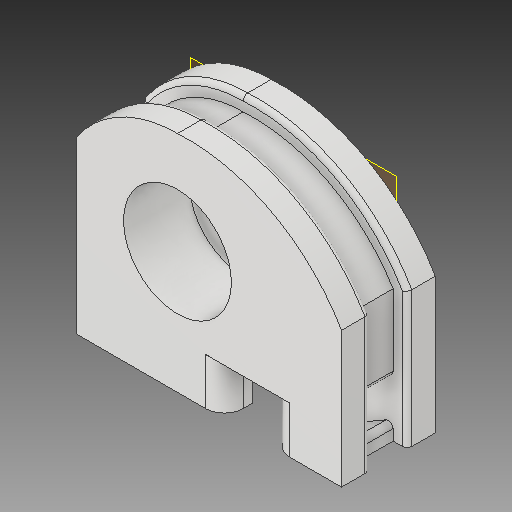
# Autodesk Inventor part: Gankenkunアンテナパーツ
Saved by Autodesk Inventor 2018 (Build 220112000, 112)
## iProperties
Category: コックピット
Created: 2018-04-09
Part Number: Gankenkunアンテナパーツ
Material: ABS プラスチック
Document SubType Name: Modeling
Designer: ito 017
Density: 1.06 g/cm^3
Appearance: 滑らか - 白
Author: ito 017
Autodesk Inventor part; units mm, degrees
ref_plane "YZ Plane" through (0, 0, 0) normal (1, 0, 0) x (0, 1, 0)
ref_plane "XZ Plane" through (0, 0, 0) normal (0, 1, 0) x (-1, 0, 0)
ref_plane "XY Plane" through (0, 0, 0) normal (0, 0, 1) x (1, 0, 0)
ref_plane "作業平面12" through (0, 0, 10) normal (0, 0, 1) x (1, 0, 0)
sketch "スケッチ48" plane through (0, 0, 10) normal (0, 0, 1) x (1, 0, 0)
  line L0 (-10.75, -3) -> (-10.75, 15.2244) projected
  line L1 (-10.75, -3) -> (17.5, -3)
  line L2 (17.5, -3) -> (17.5, 11.485)
  line L3 (-10.75, 11.485) -> (-10.75, -3)
  arc A0 (17.5, 11.485) -> (0, 20.9143) centre (1.069, 1.9444) ccw projected
  arc A1 (0, 20.9143) -> (-10.75, 15.2244) centre (0, 7.9143) ccw
  arc A2 (17.5, 11.485) -> (0, 20.9143) centre (1.069, 1.9444) ccw
  line L4 (-10.75, 15.2244) -> (-10.75, 11.485)
  circle A3 centre (0, 10) radius 3.5 projected
  circle A4 centre (0, 10) radius 3.5
  circle A5 centre (0, 10) radius 5.75
  point P0 (0, 0)
  constraints: 8 end point, 4 centre point, 4 point on circle, 2 coincident, 1 concentric, 1 horizontal, 1 parallel, 1 perpendicular, 1 vertical
extrude "押し出し40" add sketch "スケッチ48" along normal blind 10 contours L0 A1 A0 L2 L1 | A5
sketch "スケッチ50" plane through (0, 0, 20) normal (0, 0, 1) x (1, 0, 0)
  line L0 (-10.75, -3) -> (17.5, -3) projected
  line L1 (5, -3) -> (10, -3)
  line L2 (10, -3) -> (10, 2)
  line L3 (10, 2) -> (5, 2)
  line L4 (5, 2) -> (5, -3)
  line L5 (-10.75, 15.2244) -> (-10.75, -3) projected
  point P0 (0, 0)
  dimension "d179" = 15.75
  dimension "d180" = 5
  dimension "d181" = 5
  constraints: 8 end point, 2 parallel, 1 horizontal, 1 perpendicular, 1 point on line
  measures "d179" distance between parallel lines of L5 L4
  measures "d180" distance between parallel lines of L4 L2
  measures "d181" distance of L1.end L2.end
extrude "押し出し41" cut sketch "スケッチ50" against normal blind 10
sketch "スケッチ51" plane through (0, 0, 20) normal (0, 0, 1) x (1, 0, 0)
  circle A0 centre (0, 10) radius 5.75
  circle A1 centre (0, 10) radius 3.5 projected
  point P0 (0, 0)
  dimension "d184" = 11.5
  constraints: 1 centre point, 1 concentric
  measures "d184" diameter of A0
extrude "押し出し42" cut sketch "スケッチ51" against normal blind 7
sketch "スケッチ52" plane through (0, 0, 20) normal (0, 0, 1) x (1, 0, 0)
  line L0 (10, -3) -> (17.5, -3) projected
  line L1 (17.5, -3) -> (16, -3)
  line L2 (16, -3) -> (16, 11.0771)
  line L3 (16, 11.0771) -> (17.5, 11.0771)
  line L4 (17.5, 11.0771) -> (17.5, -3)
  line L5 (-10.75, -3) -> (5, -3) projected
  line L6 (-10.75, -3) -> (-9.25, -3)
  line L7 (-9.25, -3) -> (-9.25, 14.7471)
  line L8 (-9.25, 14.7471) -> (-10.75, 14.7471)
  line L9 (-10.75, 14.7471) -> (-10.75, -3)
  arc A0 (0, 20.9143) -> (-10.75, 15.2244) centre (0, 7.9143) ccw projected
  line L10 (0, 20.9143) -> (0, 19.4143)
  arc A1 (0, 19.4143) -> (-9.25, 14.7471) centre (0, 7.9143) ccw
  arc A2 (16, 11.0771) -> (0, 19.4143) centre (1.069, 1.9444) ccw
  arc A3 (17.5, 11.485) -> (0, 20.9143) centre (1.069, 1.9444) ccw projected
  line L11 (-10.75, 15.2244) -> (-10.75, 14.7471)
  line L12 (-10.75, 15.2244) -> (-10.75, -3) projected
  line L13 (17.5, -3) -> (17.5, 11.485) projected
  line L14 (17.5, 11.0771) -> (17.5, 11.485)
  point P0 (0, 0)
  dimension "d187" = 1.5
  dimension "d188" = 1.5
  dimension "d189" = 1.5
  constraints: 22 end point, 4 parallel, 4 point on circle, 2 centre point, 2 collinear, 2 concentric, 2 horizontal, 2 perpendicular, 1 vertical
  measures "d187" distance between parallel lines of L9 L7
  measures "d188" distance between parallel lines of L4 L2
  measures "d189" distance of L10.start L10.end
extrude "押し出し43" cut sketch "スケッチ52" against normal blind 7
sketch "スケッチ53" plane through (0, 0, 20) normal (0, 0, 1) x (1, 0, 0)
  line L0 (10, -3) -> (12.5, -3)
  line L1 (12.5, -3) -> (12.5, 0)
  line L2 (12.5, 0) -> (10, 0)
  line L3 (10, 0) -> (10, -3)
  line L4 (-10.75, -3) -> (5, -3) projected
  line L5 (5, -3) -> (0, -3)
  line L6 (0, -3) -> (0, -1)
  line L7 (0, -1) -> (5, -1)
  line L8 (5, -1) -> (5, -3)
  line L9 (12.5, -3) -> (16, -0.9793)
  line L10 (16, -3) -> (16, 11.0771) projected
  line L11 (10, 2) -> (10, -3) projected
  line L12 (10, -0.2865) -> (16, 3.1776)
  line L13 (10, -3) -> (16, -3) projected
  line L14 (0, -3) -> (-9.25, 2.382)
  line L15 (-9.25, 14.7471) -> (-9.25, -3) projected
  line L16 (5, -3) -> (5, 2) projected
  line L17 (5, -1.6285) -> (-9.25, 6.6628)
  point P0 (0, 0)
  dimension "d192" = 2.5
  dimension "d193" = 3
  dimension "d194" = 2
  dimension "d195" = 5
  dimension "d197" = 3.6
  dimension "d198" = 30
  dimension "d199" = 3.7
  constraints: 24 end point, 6 parallel, 6 point on line, 2 horizontal, 2 perpendicular
  measures "d192" distance of L0.start L0.end
  measures "d193" distance of L0.end L1.end
  measures "d194" distance of L5.end L6.end
  measures "d195" distance of L6.end L7.end
  measures "d197" distance between parallel lines of L9 L12
  measures "d198" angle of L13 L9
  measures "d199" distance between parallel lines of L17 L14
extrude "押し出し44" cut sketch "スケッチ53" against normal blind 7 contours L3 L12 L2 L1 L0 | L1 L2 L12 L10 L9 | L3 L2 L12 | L6 L7 L17 L8 L4 | L14 L15 L17 L7 L6 | L17 L7 L8
sketch "スケッチ54" plane through (0, 0, 20) normal (0, 0, 1) x (1, 0, 0)
  line L0 (-10.75, -3) -> (-10.75, 15.2244) projected
  line L1 (-10.75, -3) -> (-10.75, 15.2244)
  arc A0 (0, 19.4143) -> (-9.25, 14.7471) centre (0, 7.9143) ccw projected
  line L2 (-10.75, 15.2244) -> (-9.25, 14.7471)
  line L3 (-9.25, 14.7471) -> (-9.25, 6.6628) projected
  line L4 (-9.25, 14.7471) -> (-9.25, 6.6628)
  line L5 (-9.25, 6.6628) -> (3.9198, -1) projected
  line L6 (-9.25, 6.6628) -> (3.9198, -1)
  line L7 (3.9198, -1) -> (5, -1)
  line L8 (5, 2) -> (5, -3) projected
  line L9 (5, -3) -> (5, -1)
  line L10 (5, -3) -> (0, -3) projected
  line L11 (5, -3) -> (0, -3)
  line L12 (0, -3) -> (-9.25, 2.382)
  line L13 (-9.25, 2.382) -> (-9.25, -3) projected
  line L14 (-9.25, 2.382) -> (-9.25, -3)
  line L15 (-9.25, -3) -> (-10.75, -3)
  line L16 (10, -3) -> (17.5, -3) projected
  line L17 (17.5, 11.485) -> (17.5, -3) projected
  line L18 (17.5, -3) -> (17.5, 11.485)
  arc A1 (16, 11.0771) -> (0, 19.4143) centre (1.069, 1.9444) ccw projected
  line L19 (17.5, 11.485) -> (16, 11.0771)
  line L20 (16, 3.1776) -> (16, 11.0771) projected
  line L21 (16, 11.0771) -> (16, 3.1776)
  line L22 (10.4962, 0) -> (16, 3.1776) projected
  line L23 (16, 3.1776) -> (10.4962, 0)
  line L24 (10, 0) -> (10.4962, 0) projected
  line L25 (10.4962, 0) -> (10, 0)
  line L26 (10, -3) -> (10, 0) projected
  line L27 (10, 0) -> (10, -3)
  line L28 (12.5, -3) -> (10, -3) projected
  line L29 (10, -3) -> (12.5, -3)
  line L30 (16, -3) -> (16, -0.9793) projected
  line L31 (12.5, -3) -> (16, -0.9793)
  line L32 (16, -0.9793) -> (16, -3)
  line L33 (16, -3) -> (17.5, -3)
  arc A2 (0, 20.9143) -> (-10.75, 15.2244) centre (0, 7.9143) ccw projected
  arc A3 (17.5, 11.485) -> (0, 20.9143) centre (1.069, 1.9444) ccw
  arc A4 (-10.75, 0.6042) -> (-10.3133, 0) centre (0, 7.9143) ccw
  arc A5 (-9.4623, -1) -> (-9.25, -1.2201) centre (0, 7.9143) ccw
  arc A6 (10, -0.3923) -> (10.3133, 0) centre (0, 7.9143) ccw
  arc A7 (0, 19.4143) -> (-9.25, 14.7471) centre (0, 7.9143) ccw
  arc A8 (16, 11.0771) -> (0, 19.4143) centre (1.069, 1.9444) ccw
  point P0 (0, 0)
  constraints: 40 end point, 12 collinear, 12 point on circle, 7 point on line, 6 centre point, 3 concentric, 3 parallel, 3 perpendicular
extrude "押し出し45" add sketch "スケッチ54" against normal blind 3 contours L0 L2 L3 L5 L7 L8 L10 L12 L13 L15 | A2 A3 L19 A1 A0 L2 | L17 L16 L30 L31 L26 A6 L24 L22 L20 L19 | A6 L26 L24
fillet "フィレット26" radius 2 4 edges at (5, -0.5, 20) (10, -0.5, 20) (5, -0.5, 10) (10, -0.5, 10)
fillet "フィレット27" radius 0.5 12 edges at (-10.75, 6.1122, 17) (-10.75, 6.1122, 13) (-9.25, 6.6628, 15) (-9.25, 2.382, 15) (17.5, 4.2425, 13) (17.5, 4.2425, 17) (16, 3.1776, 15) (16, -0.9793, 15) (10.0815, 18.6709, 13) (10.0815, 18.6709, 17) (-6.0815, 19.4041, 17) (-6.0815, 19.4041, 13)
